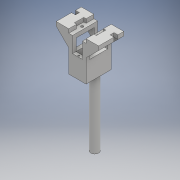
# Autodesk Inventor part: core_structure
Saved by Autodesk Inventor 2018 (Build 220112000, 112)
## iProperties
Created: 2018-02-12
Part Number: core_structure
Material: Generic
Document SubType Name: Modeling
Designer: Bardo91
Density: 1 g/cm^3
Appearance: Default
Author: Bardo91
Autodesk Inventor part; units mm, degrees
ref_plane "YZ Plane" through (0, 0, 0) normal (1, 0, 0) x (0, 1, 0)
ref_plane "XZ Plane" through (0, 0, 0) normal (0, 1, 0) x (-1, 0, 0)
ref_plane "XY Plane" through (0, 0, 0) normal (0, 0, 1) x (1, 0, 0)
sketch "Sketch1" plane through (0, 0, 0) normal (0, 0, 1) x (1, 0, 0)
  line L0 (0, 0) -> (18, 0)
  line L1 (18, 0) -> (18, 32)
  line L2 (18, 32) -> (0, 32)
  line L3 (0, 32) -> (0, 0)
  dimension "d0" = 18
  dimension "d1" = 32
  constraints: 8 end point, 2 perpendicular, 1 horizontal, 1 vertical
  measures "d0" distance of L0.start L0.end
  measures "d1" distance of L0.end L1.end
extrude "base" add sketch "Sketch1" along normal blind 25
sketch "Sketch2" plane through (0, 0, 25) normal (0, 0, 1) x (1, 0, 0)
  line L0 (18, 32) -> (0, 32) projected
  line L1 (9, 32) -> (9, 0)
  line L2 (9, 16) -> (9, 27.5)
  line L3 (9, 16) -> (20.5, 16) construction
  line L4 (9, 27.5) -> (15.25, 27.5)
  line L5 (15.25, 27.5) -> (15.25, 4.5)
  line L6 (15.25, 4.5) -> (2.75, 4.5)
  line L7 (2.75, 4.5) -> (2.75, 27.5)
  line L8 (2.75, 27.5) -> (9, 27.5)
  line L9 (0, 0) -> (18, 0) projected
  dimension "d4" = 11.5
  dimension "d5" = 90
  dimension "d6" = 6.25
  dimension "d7" = 23
  dimension "d8" = 12.5
  constraints: 16 end point, 6 perpendicular, 3 midpoint, 1 collinear, 1 horizontal, 1 point on line, 1 vertical
  measures "d4" distance of L2.start L2.end
  measures "d5" angle of L3 L2
  measures "d6" distance of L2.end L4.end
  measures "d7" distance of L4.end L5.end
  measures "d8" distance of L5.end L6.end
extrude "servo_place" cut sketch "Sketch2" against normal blind 18
sketch "Sketch4" plane through (0, 0, 0) normal (0, 0, -1) x (-1, 0, 0)
  line L0 (-18, 32) -> (0, 32) projected
  line L1 (-9, 32) -> (-9, 22)
  circle A0 centre (-9, 22) radius 5
  point P0 (0, 0)
  point P1 (-13, 32)
  point P2 (-5, 32)
  dimension "d18" = 10
  dimension "d19" = 10
  constraints: 2 end point, 1 centre point, 1 coincident, 1 midpoint, 1 vertical
  measures "d18" distance of L1.start L1.end
  measures "d19" diameter of A0
extrude "attacher" add sketch "Sketch4" along normal blind 120
fillet "Fillet2" radius 4 1 edges at (14, 22, 0)
sketch "Sketch3" plane through (0, 0, 25) normal (0, 0, 1) x (1, 0, 0)
  line L0 (2.75, 27.5) -> (15.25, 27.5) projected
  line L1 (9, 27.5) -> (9, 30.3)
  circle A0 centre (9, 30.3) radius 1
  line L2 (15.25, 4.5) -> (2.75, 4.5) projected
  line L3 (9, 4.5) -> (9, 1.7)
  circle A1 centre (9, 1.7) radius 1
  point P0 (0, 0)
  dimension "d11" = 2.8
  dimension "d12" = 2
  dimension "d13" = 2.8
  dimension "d14" = 2
  constraints: 4 end point, 2 centre point, 2 coincident, 2 midpoint, 2 vertical
  measures "d11" distance of L1.start L1.end
  measures "d12" diameter of A0
  measures "d13" distance of L3.start L3.end
  measures "d14" diameter of A1
extrude "screws_servo" cut sketch "Sketch3" against normal through all
sketch "Sketch5" plane through (9, 22, -120) normal (0, 0, -1) x (-1, 0, 0)
  circle A0 centre (0, 0) radius 2.5
  point P0 (9, -22)
  dimension "d23" = 5
  constraints: 1 centre point
  measures "d23" diameter of A0
extrude "hole_bar_rigify" cut sketch "Sketch5" against normal through all
sketch "Sketch6" plane through (0, 0, 25) normal (0, 0, 1) x (1, 0, 0)
  line L0 (0, 32) -> (0, 0) projected
  line L1 (2.75, 27.5) -> (15.25, 27.5) projected
  line L2 (0, 32) -> (2.75, 32)
  line L3 (2.75, 32) -> (2.75, 27.5)
  line L4 (2.75, 27.5) -> (0, 27.5)
  line L5 (0, 27.5) -> (0, 32)
  line L6 (18, 32) -> (15.2563, 32)
  line L7 (15.2563, 32) -> (15.2563, 27.5)
  line L8 (15.2563, 27.5) -> (18, 27.5)
  line L9 (18, 27.5) -> (18, 32)
  line L10 (15.25, 27.5) -> (15.25, 4.5) projected
  line L11 (18, 0) -> (15.25, 0)
  line L12 (15.25, 0) -> (15.25, 4.5)
  line L13 (15.25, 4.5) -> (18, 4.5)
  line L14 (18, 4.5) -> (18, 0)
  line L15 (0, 0) -> (2.75, 0)
  line L16 (2.75, 0) -> (2.75, 4.5)
  line L17 (2.75, 4.5) -> (0, 4.5)
  line L18 (0, 4.5) -> (0, 0)
  constraints: 32 end point, 8 parallel, 4 horizontal, 4 perpendicular, 4 point on line
extrude "pilars_top" add sketch "Sketch6" along normal blind 20
sketch "Sketch9" plane through (0, 0, 45) normal (0, 0, 1) x (1, 0, 0)
  line L0 (0, 32) -> (0, 22) projected
  line L1 (18, 0) -> (18, 22) projected
  line L2 (0, 32) -> (18, 32)
  line L3 (18, 32) -> (18, 0)
  line L4 (18, 0) -> (0, 0)
  line L5 (0, 0) -> (0, 32)
  line L6 (18, 32) -> (36, 32)
  line L7 (36, 32) -> (36, 0)
  line L8 (36, 0) -> (18, 0)
  line L9 (0, 32) -> (-18, 32)
  line L10 (-18, 32) -> (-18, 0)
  line L11 (-18, 0) -> (0, 0)
  point P0 (0, 0)
  dimension "d39" = 18
  dimension "d40" = 18
  constraints: 20 end point, 5 perpendicular, 3 parallel, 1 horizontal, 1 point on line, 1 vertical
  measures "d39" distance of L2.end L6.end
  measures "d40" distance of L0.start L9.end
extrude "base_top" add sketch "Sketch9" along normal blind 5
chamfer "Chamfer1" distance 18 angle 45 4 edges at (18, 2.25, 45) (18, 29.75, 45) (0, 2.25, 45) (0, 29.75, 45)
sketch "Sketch10" plane through (0, 0, 50) normal (0, 0, 1) x (1, 0, 0)
  circle A0 centre (9, 22) radius 2.5 projected
  circle A1 centre (9, 22) radius 6
  point P0 (0, 0)
  dimension "d46" = 12
  constraints: 1 centre point, 1 coincident
  measures "d46" diameter of A1
extrude "screw_hole" cut sketch "Sketch10" against normal blind 5 contours A0 | A1
sketch "Sketch11" plane through (0, 0, 50) normal (0, 0, 1) x (1, 0, 0)
  circle A0 centre (9, 22) radius 2.5 projected
  line L0 (9, 22) -> (36, 22)
  line L1 (36, 4.5) -> (36, 27.5) projected
  line L2 (36, 22) -> (36, 24.5)
  line L3 (36, 24.5) -> (31, 24.5)
  line L4 (31, 24.5) -> (31, 19.5)
  line L5 (31, 19.5) -> (36, 19.5)
  line L6 (36, 22) -> (36, 19.5)
  line L7 (9, 22) -> (-18, 22)
  line L8 (-18, 27.5) -> (-18, 4.5) projected
  line L9 (-18, 22) -> (-18, 24.5)
  line L10 (-18, 24.5) -> (-13, 24.5)
  line L11 (-13, 24.5) -> (-13, 19.5)
  line L12 (-13, 19.5) -> (-18, 19.5)
  line L13 (-18, 19.5) -> (-18, 22)
  point P0 (0, 0)
  point P1 (36, 0)
  point P2 (36, 32)
  point P3 (-18, 32)
  point P4 (-18, 0)
  dimension "d49" = 2.5
  dimension "d50" = 5
  dimension "d51" = 5
  dimension "d52" = 2.5
  dimension "d53" = 5
  dimension "d54" = 5
  constraints: 24 end point, 7 point on line, 5 perpendicular, 2 collinear, 2 horizontal
  measures "d49" distance of L0.end L2.end
  measures "d50" distance of L2.end L3.end
  measures "d51" distance of L3.end L4.end
  measures "d52" distance of L7.end L9.end
  measures "d53" distance of L9.end L10.end
  measures "d54" distance of L10.end L11.end
extrude "Extrusion11" cut sketch "Sketch11" against normal blind 5 contours L4 L3 L1 L0 | L0 L1 L5 L4 | L11 L12 L8 L7 | L7 L8 L10 L11
sketch "Boceto12" plane through (9, 22, -120) normal (0, 0, -1) x (-1, 0, 0)
  circle A0 centre (0, 0) radius 5
  point P0 (9, -22)
  constraints: 1 centre point
extrude "Extrusión12" cut sketch "Boceto12" against normal blind 30
sketch "Boceto13" plane through (0, 32, 0) normal (0, 1, 0) x (1, 0, 0)
  line L0 (2.75, -25) -> (2.75, -7) projected
  line L1 (15.25, -25) -> (15.25, -7) projected
  line L2 (2.75, -25) -> (15.25, -25)
  line L3 (2.75, -25) -> (15.25, -25) projected
  line L4 (9, -25) -> (9, -12)
  line L5 (10, -25) -> (10, 0.0515) projected
  line L6 (9, -25) -> (22, -25) construction
  line L7 (9, -12) -> (12.5, -12)
  line L8 (9, -12) -> (5.5, -12)
  line L9 (5.5, -12) -> (5, -12)
  line L10 (5, -12) -> (5, -6)
  line L11 (5, -6) -> (13, -6)
  line L12 (13, -6) -> (13, -12)
  line L13 (13, -12) -> (12.5, -12)
  point P0 (0, 0)
  dimension "d59" = 13
  dimension "d60" = 90
  dimension "d61" = 3.5
  dimension "d62" = 3.5
  dimension "d63" = 0.5
  dimension "d64" = 6
  dimension "d65" = 8
  constraints: 20 end point, 6 perpendicular, 4 horizontal, 1 midpoint, 1 parallel, 1 point on line
  measures "d59" distance of L4.start L4.end
  measures "d60" angle of L6 L4
  measures "d61" distance of L4.end L7.end
  measures "d62" distance of L4.end L8.end
  measures "d63" distance of L8.end L9.end
  measures "d64" distance of L9.end L10.end
  measures "d65" distance of L10.end L11.end
extrude "Extrusión13" cut sketch "Boceto13" against normal blind 5 contours L8 L9 L10 L11 L5 L7 | L5 L11 L12 L13 L7
move faces "Desplazar1" translate (-2, 0, 0) faces at (0, 12.1667, 8.3333)
move faces "Desplazar2" translate (2, 0, 0) faces at (18, 12.1667, 8.3333)
sketch "Boceto14" plane through (0, 0, 50) normal (0, 0, 1) x (1, 0, 0)
  line L0 (2.75, 0) -> (2.75, 4.5) projected
  line L1 (15.2563, 32) -> (15.2563, 27.5) projected
  line L2 (2.75, 32) -> (15.2563, 32)
  line L3 (2.75, 0) -> (15.25, 0) projected
  line L4 (15.2563, 0) -> (2.75, 0)
  line L5 (2.75, 0) -> (-2, 0)
  line L6 (-2, 32) -> (2.75, 32)
  line L7 (15.25, 0) -> (20, 0)
  line L8 (20, 32) -> (15.2563, 32)
  line L9 (-2, 0) -> (-2, 10)
  line L10 (-2, 10) -> (-5, 10)
  line L11 (-2, 32) -> (-2, 22)
  line L12 (-2, 22) -> (-5, 22)
  line L13 (-5, 22) -> (-5, 10)
  line L14 (20, 0) -> (20, 10)
  line L15 (20, 10) -> (23, 10)
  line L16 (23, 10) -> (23, 22)
  line L17 (23, 22) -> (20, 22)
  line L18 (20, 22) -> (20, 32)
  point P0 (0, 0)
  dimension "d74" = 4.75
  dimension "d75" = 10
  dimension "d76" = 3
  dimension "d77" = 10
  dimension "d78" = 10
  dimension "d79" = 3
  constraints: 32 end point, 6 perpendicular, 2 point on line, 1 horizontal
  measures "d74" distance of L3.end L7.end
  measures "d75" distance of L5.end L9.end
  measures "d76" distance of L9.end L10.end
  measures "d77" distance of L6.start L11.end
  measures "d78" distance of L7.end L14.end
  measures "d79" distance of L14.end L15.end
extrude "Extrusión14" cut sketch "Boceto14" against normal blind 5
sketch "Boceto15" plane through (0, 0, 45) normal (0, 0, -1) x (-1, 0, 0)
  line L0 (2, 27.5) -> (2, 22) projected
  line L1 (2, 27.5) -> (7, 27.5)
  line L2 (18, 27.5) -> (2, 27.5) projected
  line L3 (7, 27.5) -> (7, 4.5)
  line L4 (7, 4.5) -> (-2.75, 4.5)
  line L5 (2, 27.5) -> (-2.75, 27.5) projected
  line L6 (-2.75, 4.5) -> (-2.75, 27.5)
  line L7 (-2.75, 27.5) -> (2, 27.5)
  line L8 (-36, 4.5) -> (-20, 4.5) projected
  line L9 (-20, 4.5) -> (-25, 4.5)
  line L10 (-25, 4.5) -> (-25, 27.5)
  line L11 (-36, 27.5) -> (-20, 27.5) projected
  line L12 (-25, 27.5) -> (-15.2563, 27.5)
  line L13 (-15.2563, 27.5) -> (-15.2563, 4.5)
  line L14 (-20, 4.5) -> (-20, 0) projected
  line L15 (-15.2563, 4.5) -> (-20, 4.5)
  point P0 (0, 0)
  dimension "d82" = 5
  dimension "d83" = 5
  constraints: 20 end point, 6 perpendicular, 4 point on line, 1 collinear, 1 horizontal
  measures "d82" distance of L0.start L1.end
  measures "d83" distance of L8.end L9.end
extrude "Extrusión15" add sketch "Boceto15" along normal blind 5
sketch "Boceto16" plane through (0, 0, 45) normal (0, 0, 1) x (1, 0, 0)
  line L0 (-5, 22) -> (-5, 10) projected
  line L1 (-5, 16) -> (-1, 16)
  circle A0 centre (-1, 16) radius 1.5
  line L2 (23, 10) -> (23, 22) projected
  line L3 (23, 16) -> (19, 16)
  circle A1 centre (19, 16) radius 1.5
  point P0 (0, 0)
  dimension "d86" = 4
  dimension "d87" = 3
  dimension "d88" = 4
  dimension "d89" = 3
  constraints: 4 end point, 2 centre point, 2 coincident, 2 horizontal, 2 midpoint
  measures "d86" distance of L1.start L1.end
  measures "d87" diameter of A0
  measures "d88" distance of L3.start L3.end
  measures "d89" diameter of A1
extrude "Extrusión16" cut sketch "Boceto16" against normal blind 5
body "Solid1"
